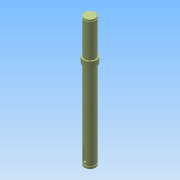
# Autodesk Inventor part: 齿轮60-2万向轴
Saved by Autodesk Inventor 2015 (Build 190159000, 159)
## iProperties
Created: 2017-05-27
Part Number: 齿轮60-2万向轴
Material: 常规
Document SubType Name: Modeling
Designer: Administrator
Density: 1 g/cm^3
Appearance: 铬酸锌 2
Author: Administrator
Autodesk Inventor part; units mm, degrees
ref_plane "YZ Plane" through (0, 0, 0) normal (1, 0, 0) x (0, 1, 0)
sketch "草图1" plane through (0, 0, 0) normal (0, 0, 1) x (1, 0, 0)
  circle A0 centre (0, 0) radius 10
  dimension "d0" = 20
  constraints: 1 centre point, 1 coincident
  measures "d0" diameter of A0
extrude "拉伸1" add sketch "草图1" along normal blind 237.2
ref_plane "工作平面1" through (0, -10, 0) normal (0, 1, 0) x (-1, 0, 0)
sketch "草图2" plane through (0, -10, 0) normal (0, 1, 0) x (-1, 0, 0)
  line L0 (3, 33.7) -> (-3, 33.7)
  line L1 (-3, 33.7) -> (-3, 11.7)
  line L2 (-3, 11.7) -> (3, 11.7)
  line L3 (3, 11.7) -> (3, 33.7)
  arc A0 (3, 33.7) -> (-3, 33.7) centre (0, 33.7) ccw
  arc A1 (-3, 11.7) -> (3, 11.7) centre (0, 11.7) ccw
  line L4 (0, 0) -> (0, 11.7)
  dimension "d3" = 6
  dimension "d4" = 22
  dimension "d5" = 11.7
  constraints: 10 end point, 4 point on circle, 4 tangent, 2 centre point, 2 parallel, 1 horizontal, 1 midpoint, 1 perpendicular, 1 vertical
  measures "d3" distance of L1.end L2.end
  measures "d4" distance of L0.end L1.end
  measures "d5" distance of L4.start L4.end
extrude "拉伸2" cut sketch "草图2" along normal blind 2.5
sketch "草图3" plane through (0, 0, 0) normal (0, 1, 0) x (-1, 0, 0)
  line L0 (-9.175, 5.2) -> (-16.1829, 5.2)
  line L1 (-16.1829, 5.2) -> (-16.1829, 4)
  line L2 (-16.1829, 4) -> (-9.175, 4)
  line L3 (-9.175, 4) -> (-9.175, 5.2)
  line L4 (0, 0) -> (0, -12.502)
  line L5 (-10, 0) -> (10, 0) projected
  dimension "d8" = 12.502
  dimension "d9" = 4
  dimension "d10" = 1.2
  dimension "d11" = 9.175
  dimension "d12" = 7.0079
  constraints: 10 end point, 2 parallel, 1 horizontal, 1 perpendicular, 1 vertical
  measures "d8" distance of L4.start L4.end
  measures "d9" distance between parallel lines of L5 L2
  measures "d10" distance of L1.end L0.end
  measures "d11" distance between parallel lines of L4 L3
  measures "d12" distance of L0.start L0.end
revolve "旋转1" cut sketch "草图3" angle 360 about axis through (0, 0, 0) along (0, 0, -1)
chamfer "倒角1" distance 0.5 angle 45 1 edges at (-10, 0, 0)
ref_plane "工作平面2" through (0, 0, 162.2) normal (0, 0, -1) x (-1, 0, 0)
sketch "草图4" plane through (0, 0, 162.2) normal (0, 0, -1) x (-1, 0, 0)
  circle A0 centre (0, 0) radius 12
  circle A1 centre (0, 0) radius 10 projected
  dimension "d18" = 24
  constraints: 1 centre point, 1 concentric
  measures "d18" diameter of A0
extrude "拉伸3" add sketch "草图4" against normal blind 10
chamfer "倒角2" distance 0.5 angle 45 1 edges at (-10, 0, 237.2)
sketch "草图5" plane through (0, 0, 0) normal (0, 1, 0) x (-1, 0, 0)
  line L0 (-12, 234.9) -> (-9.175, 234.9)
  line L1 (-9.175, 234.9) -> (-9.175, 233.7)
  line L2 (-9.175, 233.7) -> (-12, 233.7)
  line L3 (-12, 233.7) -> (-12, 234.9)
  line L4 (-9.5, 237.2) -> (9.5, 237.2) projected
  line L5 (10, 236.7) -> (-10, 236.7) projected
  line L6 (0, 236.7) -> (0, 240.4719)
  point P0 (0, 0)
  dimension "d24" = 1.2
  dimension "d25" = 2.3
  dimension "d26" = 3.7719
  dimension "d27" = 12
  dimension "d29" = 9.175
  constraints: 10 end point, 2 parallel, 1 horizontal, 1 midpoint, 1 perpendicular, 1 vertical
  measures "d24" distance of L0.end L1.end
  measures "d25" distance between parallel lines of L4 L0
  measures "d26" distance of L6.start L6.end
  measures "d27" distance between parallel lines of L6 L3
  measures "d29" distance between parallel lines of L6 L1
revolve "旋转2" cut sketch "草图5" angle 360 about axis through (0, 0, 236.7) along (0, 0, 1)
